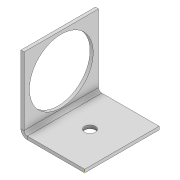
# Autodesk Inventor part: Attaching Component
Saved by Autodesk Inventor 2021 (Build 250183000, 183)
## iProperties
Created: 2021-06-28
Part Number: Attaching Component
Material: Generic
Document SubType Name: Sheet Metal
Designer: RahulRC
Density: 1 g/cm^3
Sheet Metal Rule: Default_mm
Appearance: Default
Author: RahulRC
Autodesk Inventor part; units mm, degrees
ref_plane "YZ Plane" through (0, 0, 0) normal (1, 0, 0) x (0, 1, 0)
ref_plane "XZ Plane" through (0, 0, 0) normal (0, 1, 0) x (-1, 0, 0)
ref_plane "XY Plane" through (0, 0, 0) normal (0, 0, 1) x (1, 0, 0)
sketch "Sketch1" plane through (0, 0, 0) normal (0, 1, 0) x (-1, 0, 0)
  point P0 (0, 0)
sketch "Sketch2" plane through (0, 0, 0) normal (0, 1, 0) x (-1, 0, 0)
  line L0 (0, 0) -> (0, -35)
  line L1 (0, -35) -> (30, -35)
  line L2 (30, -35) -> (30, 0)
  line L3 (30, 0) -> (0, 0)
extrude "Plate1" add sketch "Sketch2" along normal blind 1.5
sketch "Sketch3" plane through (-28.5, 0, 0) normal (-1, 0, 0) x (0, -1, 0)
  line L0 (0, -35) -> (0, 0)
  line L1 (0, 0) -> (-35, 0)
  line L2 (-35, 0) -> (-35, -35)
  line L3 (-35, -35) -> (0, -35)
  constraints: 6 end point, 1 horizontal, 1 perpendicular, 1 vertical
edge flange "Flange1" height 35 angle 90 thickness 1.5 bend radius 1.5 thickness toward (-1, 0, 0) relief tear relief width 1.5 relief depth 0.75 edges at (-30, 1.5, -17.5) wall of the first edge with corners at (-28.5, 0, -35) (-28.5, 0, 0) (-28.5, 35, 0) (-28.5, 35, -35)
bend "Bend1"
corner "Corner1"
sketch "Sketch4" plane through (-28.5, 35, 0) normal (1, 0, 0) x (0, 0, -1)
  line L0 (35, -32) -> (35, 0) projected
  line L1 (35, -33.5) -> (0, -33.5) projected
  point P0 (0, -35)
  point P1 (17.5, -16.5)
  dimension "d14" = 17.5
  dimension "d15" = 17
  measures "d14" distance from line of L0 point (17.5, -16.5)
  measures "d15" distance from line of L1 point (17.5, -16.5)
hole "Hole1" at (-28.5, 18.5, -17.5) direction (-1, 0, 0) diameter 30 depth 1.5 tip angle 120
sketch "Sketch5" plane through (0, 1.5, 0) normal (0, 1, 0) x (1, 0, 0)
  line L0 (-27, 35) -> (0, 35) projected
  line L1 (0, 35) -> (0, 0) projected
  point P0 (-15, 17.5)
  dimension "d23" = 17.5
  dimension "d24" = 15
  measures "d23" distance from line of L0 point (-15, 17.5)
  measures "d24" distance from line of L1 point (-15, 17.5)
hole "Hole2" at (-15, 1.5, -17.5) direction (0, -1, 0) diameter 5 depth 1.5 tip angle 120
equation "\"d21\" = Thickness"
equation "\"d30\" = Thickness"
equation "\"d3\" = Thickness"
equation "\"d4\" = BendReliefWidth"
equation "\"d5\" = BendReliefDepth"
equation "\"d6\" = MinimumRemnant"
equation "\"d7\" = TransitionRadius"
equation "\"d10\" = BendRadius"
equation "\"d11\" = CornerReliefSize"
equation "\"d12\" = GapSize"
equation "\"d13\" = JacobiRadiusSize"
equation "\"BendRadius\" = Thickness"
equation "\"BendReliefWidth\" = Thickness"
equation "\"BendReliefDepth\" = 0.5 * Thickness"
equation "\"CornerReliefSize\" = 4 * Thickness"
equation "\"MinimumRemnant\" = 2 * Thickness"
equation "\"TransitionRadius\" = BendRadius"
equation "\"JacobiRadiusSize\" = BendRadius"
equation "\"GapSize\" = Thickness"
equation "\"Thickness\" = 1.5"
body "Solid1"
